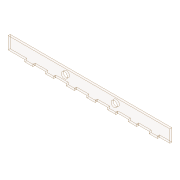
# Autodesk Inventor part: Divisória-30cm c rolamento
Saved by Autodesk Inventor 2020 (Build 240168000, 168)
## iProperties
Created: 2021-09-21
Part Number: Divisória-30cm c rolamento
Material: Generic
Document SubType Name: Modeling
Designer: pablo
Density: 1 g/cm^3
Appearance: Polycarbonate - Smoked
Author: pablo
Autodesk Inventor part; units mm, degrees
ref_plane "YZ Plane" through (0, 0, 0) normal (1, 0, 0) x (0, 1, 0)
ref_plane "XZ Plane" through (0, 0, 0) normal (0, 1, 0) x (-1, 0, 0)
ref_plane "XY Plane" through (0, 0, 0) normal (0, 0, 1) x (1, 0, 0)
sketch "Sketch1" plane through (0, 0, 0) normal (0, 0, 1) x (1, 0, 0)
  line L0 (-195, 15) -> (195, 15)
  line L1 (195, 15) -> (195, -15)
  line L2 (195, -15) -> (-195, -15)
  line L3 (-195, -15) -> (-195, 15)
  line L4 (-195, 15) -> (195, -15) construction
  line L5 (195, 15) -> (-195, -15) construction
  point P0 (0, 0)
  dimension "d0" = 390
  dimension "d1" = 30
  constraints: 12 end point, 2 midpoint, 2 parallel, 1 horizontal, 1 perpendicular
  measures "d0" distance of L1.end L2.end
  measures "d1" distance of L0.end L1.end
extrude "Base" add sketch "Sketch1" along normal blind 5
sketch "Sketch3" plane through (0, 0, 5) normal (0, 0, 1) x (1, 0, 0)
  circle A0 centre (60.7, 0) radius 7.5
  circle A1 centre (-59.3, 0) radius 7.5
  line L0 (195, -15) -> (195, 15) projected
  dimension "d16" = 15
  dimension "d17" = 15
  dimension "d20" = 134.3
  dimension "d22" = 120
  constraints: 2 centre point, 1 coincident
  measures "d16" diameter of A0
  measures "d17" diameter of A1
  measures "d20" distance from line of L0 A0.centre
  measures "d22" distance of point (-59.3, 0) A0.centre
extrude "Extrusion3" cut sketch "Sketch3" against normal blind 10
sketch "Sketch4" plane through (0, 0, 5) normal (0, 0, 1) x (1, 0, 0)
  line L0 (-195, -15) -> (195, -15) projected
  line L1 (165, -15) -> (145, -15)
  line L2 (145, -15) -> (145, -20)
  line L3 (145, -20) -> (165, -20)
  line L4 (165, -20) -> (165, -15)
  line L5 (115, -15) -> (95, -15)
  line L6 (95, -15) -> (95, -20)
  line L7 (95, -20) -> (115, -20)
  line L8 (115, -20) -> (115, -15)
  line L9 (65, -15) -> (45, -15)
  line L10 (45, -15) -> (45, -20)
  line L11 (45, -20) -> (65, -20)
  line L12 (65, -20) -> (65, -15)
  line L13 (15, -15) -> (-5, -15)
  line L14 (-5, -15) -> (-5, -20)
  line L15 (-5, -20) -> (15, -20)
  line L16 (15, -20) -> (15, -15)
  line L17 (-35, -15) -> (-55, -15)
  line L18 (-55, -15) -> (-55, -20)
  line L19 (-55, -20) -> (-35, -20)
  line L20 (-35, -20) -> (-35, -15)
  line L21 (-85, -15) -> (-105, -15)
  line L22 (-105, -15) -> (-105, -20)
  line L23 (-105, -20) -> (-85, -20)
  line L24 (-85, -20) -> (-85, -15)
  line L25 (-135, -15) -> (-155, -15)
  line L26 (-155, -15) -> (-155, -20)
  line L27 (-155, -20) -> (-135, -20)
  line L28 (-135, -20) -> (-135, -15)
  point P0 (0, 0)
  point P1 (-35, -15)
  point P2 (-55, -15)
  point P3 (-135, -15)
  point P4 (-155, -15)
  point P5 (115, -15)
  point P6 (95, -15)
  point P7 (-85, -15)
  point P8 (-105, -15)
  point P9 (65, -15)
  point P10 (45, -15)
  point P11 (15, -15)
  point P12 (-5, -15)
  point P13 (145, -15)
  dimension "d23" = 20
  dimension "d24" = 5
  dimension "d25" = 30
  dimension "d28" = 50
  constraints: 56 end point, 2 horizontal, 2 parallel, 1 perpendicular, 1 point on line, 48 other
  measures "d23" distance of L3.end L2.end
  measures "d24" distance of L2.end L1.end
  measures "d25" horizontal distance of L0.end L3.end
  measures "d28" distance of L1.start L5.start
extrude "Extrusion4" add sketch "Sketch4" against normal blind 5
body "Solid1"
